Autodesk Inventor part; units mm, degrees
(part 3 of 3)
  line L343 (-280.6004, -49.9879) -> (-282.5075, -48.0808)
  arc A136 (-304.3004, -73.6879) -> (-303.5933, -73.9808) centre (-303.5933, -72.9808) ccw
  arc A137 (-303.5933, -68.9808) -> (-304.3004, -69.2736) centre (-303.5933, -69.9808) ccw
  line L344 (-304.3004, -73.6879) -> (-306.2075, -71.7808)
  line L345 (-304.3004, -69.2736) -> (-306.2075, -71.1808)
  line L346 (-306.2075, -71.4808) -> (-306.2075, -71.7808)
  line L347 (-306.2075, -71.4808) -> (-306.2075, -71.1808)
  line L348 (-303.5933, -68.9808) -> (-286.8217, -68.9808)
  line L349 (-286.8217, -73.9808) -> (-303.5933, -73.9808)
  arc A138 (-286.1146, -69.2736) -> (-286.8217, -68.9808) centre (-286.8217, -69.9808) ccw
  line L350 (-286.1146, -69.2736) -> (-284.2075, -71.1808)
  line L351 (-284.2075, -71.4808) -> (-284.2075, -71.1808)
  line L352 (-284.2075, -71.4808) -> (-284.2075, -71.7808)
  arc A139 (-286.8217, -73.9808) -> (-286.1146, -73.6879) centre (-286.8217, -72.9808) ccw
  line L353 (-286.1146, -73.6879) -> (-284.2075, -71.7808)
  arc A140 (-98.8004, -24.0879) -> (-98.0933, -24.3808) centre (-98.0933, -23.3808) ccw
  arc A141 (-98.0933, -19.3808) -> (-98.8004, -19.6736) centre (-98.0933, -20.3808) ccw
  line L354 (-98.8004, -24.0879) -> (-100.7075, -22.1808)
  line L355 (-98.8004, -19.6736) -> (-100.7075, -21.5808)
  line L356 (-100.7075, -21.8808) -> (-100.7075, -22.1808)
  line L357 (-100.7075, -21.8808) -> (-100.7075, -21.5808)
  line L358 (-98.0933, -19.3808) -> (-81.3217, -19.3808)
  line L359 (-81.3217, -24.3808) -> (-98.0933, -24.3808)
  arc A142 (-80.6146, -19.6736) -> (-81.3217, -19.3808) centre (-81.3217, -20.3808) ccw
  line L360 (-80.6146, -19.6736) -> (-78.7075, -21.5808)
  line L361 (-78.7075, -21.8808) -> (-78.7075, -21.5808)
  line L362 (-78.7075, -21.8808) -> (-78.7075, -22.1808)
  arc A143 (-81.3217, -24.3808) -> (-80.6146, -24.0879) centre (-81.3217, -23.3808) ccw
  line L363 (-80.6146, -24.0879) -> (-78.7075, -22.1808)
  arc A144 (-98.8004, -48.8879) -> (-98.0933, -49.1808) centre (-98.0933, -48.1808) ccw
  arc A145 (-98.0933, -44.1808) -> (-98.8004, -44.4736) centre (-98.0933, -45.1808) ccw
  line L364 (-98.8004, -48.8879) -> (-100.7075, -46.9808)
  line L365 (-98.8004, -44.4736) -> (-100.7075, -46.3808)
  line L366 (-100.7075, -46.6808) -> (-100.7075, -46.9808)
  line L367 (-100.7075, -46.6808) -> (-100.7075, -46.3808)
  line L368 (-98.0933, -44.1808) -> (-81.3217, -44.1808)
  line L369 (-81.3217, -49.1808) -> (-98.0933, -49.1808)
  arc A146 (-80.6146, -44.4736) -> (-81.3217, -44.1808) centre (-81.3217, -45.1808) ccw
  line L370 (-80.6146, -44.4736) -> (-78.7075, -46.3808)
  line L371 (-78.7075, -46.6808) -> (-78.7075, -46.3808)
  line L372 (-78.7075, -46.6808) -> (-78.7075, -46.9808)
  arc A147 (-81.3217, -49.1808) -> (-80.6146, -48.8879) centre (-81.3217, -48.1808) ccw
  line L373 (-80.6146, -48.8879) -> (-78.7075, -46.9808)
  arc A148 (-99.9004, -43.3736) -> (-99.6075, -42.6665) centre (-100.6075, -42.6665) ccw
  arc A149 (-104.6075, -42.6665) -> (-104.3146, -43.3736) centre (-103.6075, -42.6665) ccw
  line L374 (-99.9004, -43.3736) -> (-101.8075, -45.2808)
  line L375 (-104.3146, -43.3736) -> (-102.4075, -45.2808)
  line L376 (-102.1075, -45.2808) -> (-101.8075, -45.2808)
  line L377 (-102.1075, -45.2808) -> (-102.4075, -45.2808)
  line L378 (-104.6075, -42.6665) -> (-104.6075, -25.895)
  line L379 (-99.6075, -25.895) -> (-99.6075, -42.6665)
  arc A150 (-104.3146, -25.1879) -> (-104.6075, -25.895) centre (-103.6075, -25.895) ccw
  line L380 (-104.3146, -25.1879) -> (-102.4075, -23.2808)
  line L381 (-102.1075, -23.2808) -> (-102.4075, -23.2808)
  line L382 (-102.1075, -23.2808) -> (-101.8075, -23.2808)
  arc A151 (-99.6075, -25.895) -> (-99.9004, -25.1879) centre (-100.6075, -25.895) ccw
  line L383 (-99.9004, -25.1879) -> (-101.8075, -23.2808)
  arc A152 (-99.9004, -68.1736) -> (-99.6075, -67.4665) centre (-100.6075, -67.4665) ccw
  arc A153 (-104.6075, -67.4665) -> (-104.3146, -68.1736) centre (-103.6075, -67.4665) ccw
  line L384 (-99.9004, -68.1736) -> (-101.8075, -70.0808)
  line L385 (-104.3146, -68.1736) -> (-102.4075, -70.0808)
  line L386 (-102.1075, -70.0808) -> (-101.8075, -70.0808)
  line L387 (-102.1075, -70.0808) -> (-102.4075, -70.0808)
  line L388 (-104.6075, -67.4665) -> (-104.6075, -50.695)
  line L389 (-99.6075, -50.695) -> (-99.6075, -67.4665)
  arc A154 (-104.3146, -49.9879) -> (-104.6075, -50.695) centre (-103.6075, -50.695) ccw
  line L390 (-104.3146, -49.9879) -> (-102.4075, -48.0808)
  line L391 (-102.1075, -48.0808) -> (-102.4075, -48.0808)
  line L392 (-102.1075, -48.0808) -> (-101.8075, -48.0808)
  arc A155 (-99.6075, -50.695) -> (-99.9004, -49.9879) centre (-100.6075, -50.695) ccw
  line L393 (-99.9004, -49.9879) -> (-101.8075, -48.0808)
  arc A156 (-75.1004, -43.3736) -> (-74.8075, -42.6665) centre (-75.8075, -42.6665) ccw
  arc A157 (-79.8075, -42.6665) -> (-79.5146, -43.3736) centre (-78.8075, -42.6665) ccw
  line L394 (-75.1004, -43.3736) -> (-77.0075, -45.2808)
  line L395 (-79.5146, -43.3736) -> (-77.6075, -45.2808)
  line L396 (-77.3075, -45.2808) -> (-77.0075, -45.2808)
  line L397 (-77.3075, -45.2808) -> (-77.6075, -45.2808)
  line L398 (-79.8075, -42.6665) -> (-79.8075, -25.895)
  line L399 (-74.8075, -25.895) -> (-74.8075, -42.6665)
  arc A158 (-79.5146, -25.1879) -> (-79.8075, -25.895) centre (-78.8075, -25.895) ccw
  line L400 (-79.5146, -25.1879) -> (-77.6075, -23.2808)
  line L401 (-77.3075, -23.2808) -> (-77.6075, -23.2808)
  line L402 (-77.3075, -23.2808) -> (-77.0075, -23.2808)
  arc A159 (-74.8075, -25.895) -> (-75.1004, -25.1879) centre (-75.8075, -25.895) ccw
  line L403 (-75.1004, -25.1879) -> (-77.0075, -23.2808)
  arc A160 (-75.1004, -68.1736) -> (-74.8075, -67.4665) centre (-75.8075, -67.4665) ccw
  arc A161 (-79.8075, -67.4665) -> (-79.5146, -68.1736) centre (-78.8075, -67.4665) ccw
  line L404 (-75.1004, -68.1736) -> (-77.0075, -70.0808)
  line L405 (-79.5146, -68.1736) -> (-77.6075, -70.0808)
  line L406 (-77.3075, -70.0808) -> (-77.0075, -70.0808)
  line L407 (-77.3075, -70.0808) -> (-77.6075, -70.0808)
  line L408 (-79.8075, -67.4665) -> (-79.8075, -50.695)
  line L409 (-74.8075, -50.695) -> (-74.8075, -67.4665)
  arc A162 (-79.5146, -49.9879) -> (-79.8075, -50.695) centre (-78.8075, -50.695) ccw
  line L410 (-79.5146, -49.9879) -> (-77.6075, -48.0808)
  line L411 (-77.3075, -48.0808) -> (-77.6075, -48.0808)
  line L412 (-77.3075, -48.0808) -> (-77.0075, -48.0808)
  arc A163 (-74.8075, -50.695) -> (-75.1004, -49.9879) centre (-75.8075, -50.695) ccw
  line L413 (-75.1004, -49.9879) -> (-77.0075, -48.0808)
  arc A164 (-98.8004, -73.6879) -> (-98.0933, -73.9808) centre (-98.0933, -72.9808) ccw
  arc A165 (-98.0933, -68.9808) -> (-98.8004, -69.2736) centre (-98.0933, -69.9808) ccw
  line L414 (-98.8004, -73.6879) -> (-100.7075, -71.7808)
  line L415 (-98.8004, -69.2736) -> (-100.7075, -71.1808)
  line L416 (-100.7075, -71.4808) -> (-100.7075, -71.7808)
  line L417 (-100.7075, -71.4808) -> (-100.7075, -71.1808)
  line L418 (-98.0933, -68.9808) -> (-81.3217, -68.9808)
  line L419 (-81.3217, -73.9808) -> (-98.0933, -73.9808)
  arc A166 (-80.6146, -69.2736) -> (-81.3217, -68.9808) centre (-81.3217, -69.9808) ccw
  line L420 (-80.6146, -69.2736) -> (-78.7075, -71.1808)
  line L421 (-78.7075, -71.4808) -> (-78.7075, -71.1808)
  line L422 (-78.7075, -71.4808) -> (-78.7075, -71.7808)
  arc A167 (-81.3217, -73.9808) -> (-80.6146, -73.6879) centre (-81.3217, -72.9808) ccw
  line L423 (-80.6146, -73.6879) -> (-78.7075, -71.7808)
  line L424 (-235.0075, -35.3808) -> (-234.0075, -35.3808)
  line L425 (-234.0075, -35.3808) -> (-232.0075, -37.3808)
  line L426 (-232.0075, -37.3808) -> (-232.0075, -38.3808)
  line L427 (-232.0075, -38.3808) -> (-234.0075, -40.3808)
  line L428 (-234.0075, -40.3808) -> (-235.0075, -40.3808)
  line L429 (-235.0075, -40.3808) -> (-237.0075, -38.3808)
  line L430 (-237.0075, -38.3808) -> (-237.0075, -37.3808)
  line L431 (-237.0075, -37.3808) -> (-235.0075, -35.3808)
  line L432 (-235.0075, -55.3808) -> (-234.0075, -55.3808)
  line L433 (-234.0075, -55.3808) -> (-232.0075, -57.3808)
  line L434 (-232.0075, -57.3808) -> (-232.0075, -58.3808)
  line L435 (-232.0075, -58.3808) -> (-234.0075, -60.3808)
  line L436 (-234.0075, -60.3808) -> (-235.0075, -60.3808)
  line L437 (-235.0075, -60.3808) -> (-237.0075, -58.3808)
  line L438 (-237.0075, -58.3808) -> (-237.0075, -57.3808)
  line L439 (-237.0075, -57.3808) -> (-235.0075, -55.3808)
  line L440 (-150.9075, -35.3808) -> (-149.9075, -35.3808)
  line L441 (-149.9075, -35.3808) -> (-147.9075, -37.3808)
  line L442 (-147.9075, -37.3808) -> (-147.9075, -38.3808)
  line L443 (-147.9075, -38.3808) -> (-149.9075, -40.3808)
  line L444 (-149.9075, -40.3808) -> (-150.9075, -40.3808)
  line L445 (-150.9075, -40.3808) -> (-152.9075, -38.3808)
  line L446 (-152.9075, -38.3808) -> (-152.9075, -37.3808)
  line L447 (-152.9075, -37.3808) -> (-150.9075, -35.3808)
  line L448 (-150.9075, -55.3808) -> (-149.9075, -55.3808)
  line L449 (-149.9075, -55.3808) -> (-147.9075, -57.3808)
  line L450 (-147.9075, -57.3808) -> (-147.9075, -58.3808)
  line L451 (-147.9075, -58.3808) -> (-149.9075, -60.3808)
  line L452 (-149.9075, -60.3808) -> (-150.9075, -60.3808)
  line L453 (-150.9075, -60.3808) -> (-152.9075, -58.3808)
  line L454 (-152.9075, -58.3808) -> (-152.9075, -57.3808)
  line L455 (-152.9075, -57.3808) -> (-150.9075, -55.3808)
  arc A168 (-332.7004, -49.0879) -> (-331.9933, -49.3808) centre (-331.9933, -48.3808) ccw
  arc A169 (-331.9933, -44.3808) -> (-332.7004, -44.6736) centre (-331.9933, -45.3808) ccw
  line L456 (-332.7004, -49.0879) -> (-334.6075, -47.1808)
  line L457 (-334.6075, -46.8808) -> (-334.6075, -46.5808)
  line L458 (-334.6075, -46.8808) -> (-334.6075, -47.1808)
  line L459 (-332.7004, -44.6736) -> (-334.6075, -46.5808)
  line L460 (-331.9933, -44.3808) -> (-321.2217, -44.3808)
  line L461 (-321.2217, -49.3808) -> (-331.9933, -49.3808)
  arc A170 (-320.5146, -44.6736) -> (-321.2217, -44.3808) centre (-321.2217, -45.3808) ccw
  arc A171 (-321.2217, -49.3808) -> (-320.5146, -49.0879) centre (-321.2217, -48.3808) ccw
  line L462 (-320.5146, -49.0879) -> (-318.6075, -47.1808)
  line L463 (-318.6075, -46.8808) -> (-318.6075, -47.1808)
  line L464 (-318.6075, -46.8808) -> (-318.6075, -46.5808)
  line L465 (-320.5146, -44.6736) -> (-318.6075, -46.5808)
  arc A172 (-333.4004, -43.9736) -> (-333.1075, -43.2665) centre (-334.1075, -43.2665) ccw
  arc A173 (-338.1075, -43.2665) -> (-337.8146, -43.9736) centre (-337.1075, -43.2665) ccw
  line L466 (-333.4004, -43.9736) -> (-335.3075, -45.8808)
  line L467 (-335.6075, -45.8808) -> (-335.9075, -45.8808)
  line L468 (-335.6075, -45.8808) -> (-335.3075, -45.8808)
  line L469 (-337.8146, -43.9736) -> (-335.9075, -45.8808)
  line L470 (-338.1075, -43.2665) -> (-338.1075, -32.495)
  line L471 (-333.1075, -32.495) -> (-333.1075, -43.2665)
  arc A174 (-337.8146, -31.7879) -> (-338.1075, -32.495) centre (-337.1075, -32.495) ccw
  arc A175 (-333.1075, -32.495) -> (-333.4004, -31.7879) centre (-334.1075, -32.495) ccw
  line L472 (-333.4004, -31.7879) -> (-335.3075, -29.8808)
  line L473 (-335.6075, -29.8808) -> (-335.3075, -29.8808)
  line L474 (-335.6075, -29.8808) -> (-335.9075, -29.8808)
  line L475 (-337.8146, -31.7879) -> (-335.9075, -29.8808)
  arc A176 (-350.7004, -49.0879) -> (-349.9933, -49.3808) centre (-349.9933, -48.3808) ccw
  arc A177 (-349.9933, -44.3808) -> (-350.7004, -44.6736) centre (-349.9933, -45.3808) ccw
  line L476 (-350.7004, -49.0879) -> (-352.6075, -47.1808)
  line L477 (-352.6075, -46.8808) -> (-352.6075, -46.5808)
  line L478 (-352.6075, -46.8808) -> (-352.6075, -47.1808)
  line L479 (-350.7004, -44.6736) -> (-352.6075, -46.5808)
  line L480 (-349.9933, -44.3808) -> (-339.2217, -44.3808)
  line L481 (-339.2217, -49.3808) -> (-349.9933, -49.3808)
  arc A178 (-338.5146, -44.6736) -> (-339.2217, -44.3808) centre (-339.2217, -45.3808) ccw
  arc A179 (-339.2217, -49.3808) -> (-338.5146, -49.0879) centre (-339.2217, -48.3808) ccw
  line L482 (-338.5146, -49.0879) -> (-336.6075, -47.1808)
  line L483 (-336.6075, -46.8808) -> (-336.6075, -47.1808)
  line L484 (-336.6075, -46.8808) -> (-336.6075, -46.5808)
  line L485 (-338.5146, -44.6736) -> (-336.6075, -46.5808)
  arc A180 (-333.4004, -61.9736) -> (-333.1075, -61.2665) centre (-334.1075, -61.2665) ccw
  arc A181 (-338.1075, -61.2665) -> (-337.8146, -61.9736) centre (-337.1075, -61.2665) ccw
  line L486 (-333.4004, -61.9736) -> (-335.3075, -63.8808)
  line L487 (-335.6075, -63.8808) -> (-335.9075, -63.8808)
  line L488 (-335.6075, -63.8808) -> (-335.3075, -63.8808)
  line L489 (-337.8146, -61.9736) -> (-335.9075, -63.8808)
  line L490 (-338.1075, -61.2665) -> (-338.1075, -50.495)
  line L491 (-333.1075, -50.495) -> (-333.1075, -61.2665)
  arc A182 (-337.8146, -49.7879) -> (-338.1075, -50.495) centre (-337.1075, -50.495) ccw
  arc A183 (-333.1075, -50.495) -> (-333.4004, -49.7879) centre (-334.1075, -50.495) ccw
  line L492 (-333.4004, -49.7879) -> (-335.3075, -47.8808)
  line L493 (-335.6075, -47.8808) -> (-335.3075, -47.8808)
  line L494 (-335.6075, -47.8808) -> (-335.9075, -47.8808)
  line L495 (-337.8146, -49.7879) -> (-335.9075, -47.8808)
  arc A184 (-359.2004, -33.0879) -> (-358.4933, -33.3808) centre (-358.4933, -32.3808) ccw
  arc A185 (-358.4933, -28.3808) -> (-359.2004, -28.6736) centre (-358.4933, -29.3808) ccw
  line L496 (-359.2004, -33.0879) -> (-361.1075, -31.1808)
  line L497 (-361.1075, -30.8808) -> (-361.1075, -30.5808)
  line L498 (-361.1075, -30.8808) -> (-361.1075, -31.1808)
  line L499 (-359.2004, -28.6736) -> (-361.1075, -30.5808)
  line L500 (-358.4933, -28.3808) -> (-347.7217, -28.3808)
  line L501 (-347.7217, -33.3808) -> (-358.4933, -33.3808)
  arc A186 (-347.0146, -28.6736) -> (-347.7217, -28.3808) centre (-347.7217, -29.3808) ccw
  arc A187 (-347.7217, -33.3808) -> (-347.0146, -33.0879) centre (-347.7217, -32.3808) ccw
  line L502 (-347.0146, -33.0879) -> (-345.1075, -31.1808)
  line L503 (-345.1075, -30.8808) -> (-345.1075, -31.1808)
  line L504 (-345.1075, -30.8808) -> (-345.1075, -30.5808)
  line L505 (-347.0146, -28.6736) -> (-345.1075, -30.5808)
  arc A188 (-376.2004, -33.0879) -> (-375.4933, -33.3808) centre (-375.4933, -32.3808) ccw
  arc A189 (-375.4933, -28.3808) -> (-376.2004, -28.6736) centre (-375.4933, -29.3808) ccw
  line L506 (-376.2004, -33.0879) -> (-378.1075, -31.1808)
  line L507 (-378.1075, -30.8808) -> (-378.1075, -30.5808)
  line L508 (-378.1075, -30.8808) -> (-378.1075, -31.1808)
  line L509 (-376.2004, -28.6736) -> (-378.1075, -30.5808)
  line L510 (-375.4933, -28.3808) -> (-364.7217, -28.3808)
  line L511 (-364.7217, -33.3808) -> (-375.4933, -33.3808)
  arc A190 (-364.0146, -28.6736) -> (-364.7217, -28.3808) centre (-364.7217, -29.3808) ccw
  arc A191 (-364.7217, -33.3808) -> (-364.0146, -33.0879) centre (-364.7217, -32.3808) ccw
  line L512 (-364.0146, -33.0879) -> (-362.1075, -31.1808)
  line L513 (-362.1075, -30.8808) -> (-362.1075, -31.1808)
  line L514 (-362.1075, -30.8808) -> (-362.1075, -30.5808)
  line L515 (-364.0146, -28.6736) -> (-362.1075, -30.5808)
  arc A192 (-359.4004, -46.4879) -> (-359.1075, -45.7808) centre (-360.1075, -45.7808) ccw
  arc A193 (-364.1075, -45.7808) -> (-363.8146, -46.4879) centre (-363.1075, -45.7808) ccw
  line L516 (-359.4004, -46.4879) -> (-361.3075, -48.395)
  line L517 (-361.6075, -48.395) -> (-361.9075, -48.395)
  line L518 (-361.6075, -48.395) -> (-361.3075, -48.395)
  line L519 (-363.8146, -46.4879) -> (-361.9075, -48.395)
  line L520 (-364.1075, -45.7808) -> (-364.1075, -35.0092)
  line L521 (-359.1075, -35.0092) -> (-359.1075, -45.7808)
  arc A194 (-363.8146, -34.3021) -> (-364.1075, -35.0092) centre (-363.1075, -35.0092) ccw
  arc A195 (-359.1075, -35.0092) -> (-359.4004, -34.3021) centre (-360.1075, -35.0092) ccw
  line L522 (-359.4004, -34.3021) -> (-361.3075, -32.395)
  line L523 (-361.6075, -32.395) -> (-361.3075, -32.395)
  line L524 (-361.6075, -32.395) -> (-361.9075, -32.395)
  line L525 (-363.8146, -34.3021) -> (-361.9075, -32.395)
  arc A196 (-359.4004, -62.9879) -> (-359.1075, -62.2808) centre (-360.1075, -62.2808) ccw
  arc A197 (-364.1075, -62.2808) -> (-363.8146, -62.9879) centre (-363.1075, -62.2808) ccw
  line L526 (-359.4004, -62.9879) -> (-361.3075, -64.895)
  line L527 (-361.6075, -64.895) -> (-361.9075, -64.895)
  line L528 (-361.6075, -64.895) -> (-361.3075, -64.895)
  line L529 (-363.8146, -62.9879) -> (-361.9075, -64.895)
  line L530 (-364.1075, -62.2808) -> (-364.1075, -51.5092)
  line L531 (-359.1075, -51.5092) -> (-359.1075, -62.2808)
  arc A198 (-363.8146, -50.8021) -> (-364.1075, -51.5092) centre (-363.1075, -51.5092) ccw
  arc A199 (-359.1075, -51.5092) -> (-359.4004, -50.8021) centre (-360.1075, -51.5092) ccw
  line L532 (-359.4004, -50.8021) -> (-361.3075, -48.895)
  line L533 (-361.6075, -48.895) -> (-361.3075, -48.895)
  line L534 (-361.6075, -48.895) -> (-361.9075, -48.895)
  line L535 (-363.8146, -50.8021) -> (-361.9075, -48.895)
  point P0 (0, 0)
  dimension "d525" = 8
  dimension "d526" = 7.4
  dimension "d527" = 26
  dimension "d528" = 14.7
  dimension "d529" = 12
extrude "Extrusion3" cut sketch "Sketch5" against normal blind 3
body "Solid1"
